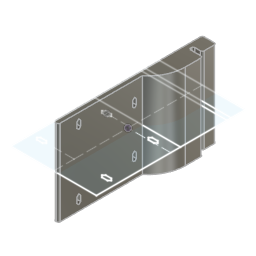
RailSlidingPlatform (Autodesk Fusion 360 design; units mm, degrees)
part number: BalconyLightsPlatformForCOPAL
Autodesk Fusion 360 part; units mm, degrees
sketch "Sketch1" plane through (0, 0, 0) normal (0, 0, 1) x (1, 0, 0) in component "BalconyLightsPlatformForCOPAL"
  line L0 (46, -80) -> (-46, -80)
  line L1 (-46, -80) -> (-46, 80)
  line L2 (-46, 80) -> (46, 80)
  line L3 (46, 80) -> (46, -80)
  line L4 (-46, 65) -> (46, 65)
  line L5 (46, 60.5) -> (-46, 60.5)
  line L6 (0, -80) -> (0, -58) construction
  line L7 (0, -58) -> (-35, -58) construction
  line L8 (-32, -60) -> (-38, -60)
  line L9 (-38, -56) -> (-32, -56)
  line L10 (-30, -58) -> (-32, -56)
  line L11 (-30, -58) -> (-32, -60)
  line L12 (-35, -58) -> (-40, -58) construction
  line L13 (-40, -58) -> (-38, -56)
  line L14 (-40, -58) -> (-38, -60)
  line L15 (0, -58) -> (0, 2) construction
  line L16 (0, 2) -> (-25, 2) construction
  line L17 (-22, 0) -> (-28, 0)
  line L18 (-28, 4) -> (-22, 4)
  line L19 (-30, 2) -> (-28, 4)
  line L20 (-30, 2) -> (-28, 0)
  line L21 (-20, 2) -> (-22, 4)
  line L22 (-20, 2) -> (-22, 0)
  line L23 (-35, -56) -> (-35, -60) construction
  line L24 (-25, 4) -> (-25, 0) construction
  line L25 (-30, 2) -> (-25, 2) construction
  line L26 (46, 0) -> (0, 0) construction
  line L27 (0, 80) -> (0, 0) construction
  line L28 (-46, 10.5) -> (46, 10.5)
  line L29 (22, 0) -> (28, 0)
  line L30 (20, 2) -> (22, 0)
  line L31 (20, 2) -> (22, 4)
  line L32 (28, 4) -> (22, 4)
  line L33 (30, 2) -> (28, 4)
  line L34 (30, 2) -> (28, 0)
  line L35 (38, -56) -> (32, -56)
  line L36 (30, -58) -> (32, -56)
  line L37 (30, -58) -> (32, -60)
  line L38 (32, -60) -> (38, -60)
  line L39 (40, -58) -> (38, -60)
  line L40 (40, -58) -> (38, -56)
  point P0 (-25, 2)
  dimension "d1" = 92
  dimension "d2" = 160
  dimension "d6" = 22
  dimension "d14" = 60
  dimension "d15" = 25
  dimension "d35" = 15
  dimension "d36" = 4.5
  dimension "d41" = 10
  dimension "d42" = 4
  dimension "d44" = 35
  dimension "d45" = 10
  dimension "d47" = 4
  dimension "d51" = 50
  constraint horizontal L0
  constraint perpendicular L0 L1
  constraint parallel L0 L2
  constraint parallel L1 L3
  constraint coincident L26.end L27.end
  constraint horizontal L4
  constraint horizontal L5
  constraint midpoint L0 L6.start
  constraint perpendicular L0 L6
  constraint perpendicular L6 L7
  constraint horizontal L8
  constraint parallel L8 L9
  constraint perpendicular L15 L16
  constraint horizontal L17
  constraint parallel L17 L18
  constraint coincident P0 L16.end
  constraint parallel L20 L21
  constraint horizontal L16
  constraint coincident L1 L5.end
  constraint coincident L1 L4.start
  constraint coincident L3 L4.end
  constraint equal L13 L14
  constraint equal L10 L11
  constraint midpoint L9 L23.start
  constraint midpoint L8 L23.end
  constraint coincident L7.end L23
  constraint collinear L7 L12
  constraint equal L19 L20
  constraint coincident L16 L21.start
  constraint equal L21 L22
  constraint midpoint L18 L24.start
  constraint midpoint L17 L24.end
  constraint coincident P0 L24
  constraint perpendicular L19 L20
  constraint perpendicular L21 L22
  constraint perpendicular L13 L14
  constraint perpendicular L10 L11
  constraint perpendicular L18 L24
  constraint equal L8 L9
  constraint midpoint L3 L26.start
  constraint midpoint L2 L27.start
  constraint perpendicular L26 L27
  constraint perpendicular L2 L27
  constraint perpendicular L9 L23
  constraint coincident L1 L28.start
  constraint coincident L3 L28.end
  constraint perpendicular L3 L28
  constraint coincident L3 L5.start
  constraint coincident L7.end L12.start
  constraint symmetric L10.start L27 L36.start
  constraint symmetric L9.end L27 L35.end
  constraint symmetric L8.start L27 L37.end
  constraint symmetric L12.end L27 L39.start
  constraint symmetric L9.start L27 L35.start
  constraint symmetric L8.end L27 L38.end
  constraint symmetric L19.start L27 L33.start
  constraint symmetric L18.start L27 L32.start
  constraint symmetric L17.end L27 L29.end
  constraint symmetric L21.start L27 L30.start
  constraint symmetric L18.end L27 L31.end
  constraint symmetric L17.start L27 L29.start
  measures "d1" distance of L1.end L2.end
  measures "d2" distance of L0.end L1.end
  measures "d6" distance of L6.start L6.end
  measures "d14" distance of L6.end L15.end
  measures "d15" distance of L15.end P0
  measures "d35" distance of L1.end L4.start
  measures "d36" distance of L4 L5
  measures "d41" distance of L10.start L12.end
  measures "d42" distance of L8 L9
  measures "d44" distance of L6.end L7.end
  measures "d45" distance of L19.start L21.start
  measures "d47" distance of L17 L18
  measures "d51" distance of L5 L28
extrude "Extrude5" add sketch "Sketch1" along normal blind 5 in component "BalconyLightsPlatformForCOPAL"
extrude "Extrude6" add sketch "Sketch1" along normal blind 15 contours L1 L2 L3 L4 in component "BalconyLightsPlatformForCOPAL"
extrude "Extrude7" add sketch "Sketch1" along normal blind 20 contours L1 L3 L5 L28 in component "BalconyLightsPlatformForCOPAL"
fillet "Fillet2" radius 2 2 edges at (0, 60.5, 5) (0, 65, 5) in component "BalconyLightsPlatformForCOPAL"
fillet "Fillet3" radius 40 1 edges at (0, 10.5, 20) in component "BalconyLightsPlatformForCOPAL"
fillet "Fillet4" radius 2 6 edges at (0, 60.5, 20) (0, 65, 15) (0, 80, 15) (0, 80, 0) (0, -80, 0) (0, -80, 5) in component "BalconyLightsPlatformForCOPAL"
move_body "Move1" bodies 1 to x (0, 0, -1) y (0, 1, 0) z (1, 0, 0) at (0, 0, 0) in component "BalconyLightsPlatformForCOPAL"
component "BalconyLightsPlatformForCOPAL" placed x (1, 0, 0) y (0, 1, 0) z (0, 0, 1) at (0, 0, 0)
